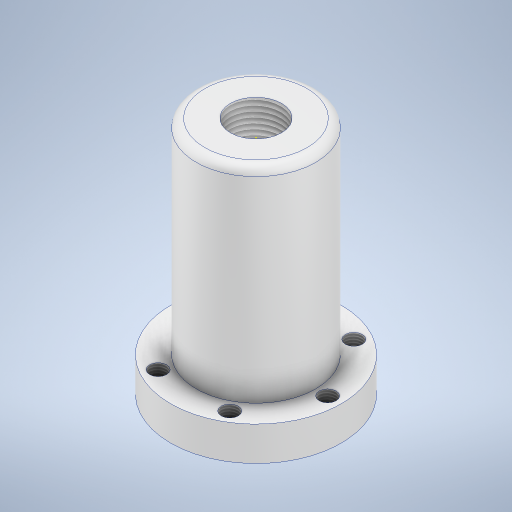
# Autodesk Inventor part: pintle body
Saved by Autodesk Inventor 2023 (Build 270158000, 158)
## iProperties
Created: 2022-07-06
Part Number: pintle body
Material: Aluminum 6061
Document SubType Name: Modeling
Designer: pc
Density: 2.7 g/cm^3
Appearance: Aluminum - Flat
Mass: 267.767 g
Surface Area: 216.281 cm^2
Volume: 99.1731 cm^3
Author: pc
Autodesk Inventor part; units mm, degrees
ref_plane "YZ Plane" through (0, 0, 0) normal (1, 0, 0) x (0, 1, 0)
sketch "Sketch1" plane through (0, 0, 0) normal (0, 1, 0) x (-1, 0, 0)
  circle A0 centre (0, 0) radius 25
  circle A1 centre (0, -30) radius 5
  circle A2 centre (30, 0) radius 5
  circle A3 centre (0, 30) radius 5
  circle A4 centre (-30, 0) radius 5
  dimension "d0" = 50
  dimension "d1" = 10
  dimension "d2" = 30
  dimension "d5" = 360
  constraints: 5 centre point, 1 coincident, 9 other
  measures "d0" diameter of A0
  measures "d1" diameter of A1
  measures "d2" distance of A1.centre point (0, 0)
extrude "Extrusion1" add sketch "Sketch1" along normal blind 10 contours A0
thread "Thread1" size "M10x1.5" class "6H" standard "ANSI Metric M Profile" length 20
thread "Thread2" size "M10x1.5" class "6H" standard "ANSI Metric M Profile" length 20
thread "Thread3" size "M10x1.5" class "6H" standard "ANSI Metric M Profile" length 20
thread "Thread4" size "M10x1.5" class "6H" standard "ANSI Metric M Profile" length 20
sketch "Sketch2" plane through (0, 10, 0) normal (0, 1, 0) x (1, 0, 0)
  circle A0 centre (0, 0) radius 17.5
  dimension "d17" = 35
  constraints: 1 centre point, 1 coincident
  measures "d17" diameter of A0
extrude "Extrusion2" add sketch "Sketch2" along normal blind 60
sketch "Sketch3" plane through (0, 70, 0) normal (0, 1, 0) x (1, 0, 0)
  circle A0 centre (0, 0) radius 10
  dimension "d20" = 20
  constraints: 1 centre point, 1 coincident
  measures "d20" diameter of A0
hole "Hole1" at (0, 70, 0) direction (0, -1, 0) diameter 8 end through all
ref_plane "Work Plane1" through (0, 68, 0) normal (0, 1, 0) x (-1, 0, 0)
ref_plane "Work Plane2" through (0, 65, 0) normal (0, -1, 0) x (1, 0, 0)
sketch "Sketch6" plane through (0, 65, 0) normal (0, -1, 0) x (1, 0, 0)
  point P0 (0, 0)
fillet "Fillet2" radius 2.5 1 edges at (-17.5, 70, 0)
thread "Thread10" size "M15x1.5" class "6H" standard "ANSI Metric M Profile" length 16.401
sketch "Sketch9" plane through (0, 70, 0) normal (0, 1, 0) x (1, 0, 0)
  circle A0 centre (0, 0) radius 4 projected
  circle A1 centre (0, 0) radius 7.5
  dimension "d61" = 15
  constraints: 1 centre point, 1 coincident
  measures "d61" diameter of A1
hole "Hole3" at (0, 70, 0) direction (0, -1, 0) diameter 15 depth 15 tip angle 118
thread "Thread11" size "M15x1.5" class "6H" standard "ANSI Metric M Profile" full length
sketch "Sketch10" plane through (0, 0, 0) normal (0, -1, 0) x (1, 0, 0)
  circle A0 centre (-21, 0) radius 2.75
  circle A1 centre (-10.5, -18.1865) radius 2.75
  circle A2 centre (10.5, -18.1865) radius 2.75
  circle A3 centre (21, 0) radius 2.75
  circle A4 centre (10.5, 18.1865) radius 2.75
  circle A5 centre (-10.5, 18.1865) radius 2.75
  point P0 (0, 0)
  dimension "d71" = 5.5
  dimension "d72" = 21
  dimension "d75" = 360
  constraints: 6 centre point, 13 other
  measures "d71" diameter of A0
  measures "d72" distance of A0.centre point (0, 0)
hole "Hole4" at (-21, 0, 0) at (-10.5, 0, 18.1865) at (10.5, 0, 18.1865) at (21, 0, 0) at (10.5, 0, -18.1865) at (-10.5, 0, -18.1865) direction (0, 1, 0) diameter 5 depth 10 tip angle 118
thread "Thread12" size "M5x0.8" class "6H" standard "ANSI Metric M Profile" full length
thread "Thread13" size "M5x0.8" class "6H" standard "ANSI Metric M Profile" full length
thread "Thread14" size "M5x0.8" class "6H" standard "ANSI Metric M Profile" full length
thread "Thread15" size "M5x0.8" class "6H" standard "ANSI Metric M Profile" full length
thread "Thread16" size "M5x0.8" class "6H" standard "ANSI Metric M Profile" full length
thread "Thread17" size "M5x0.8" class "6H" standard "ANSI Metric M Profile" full length
body "Solid1"
